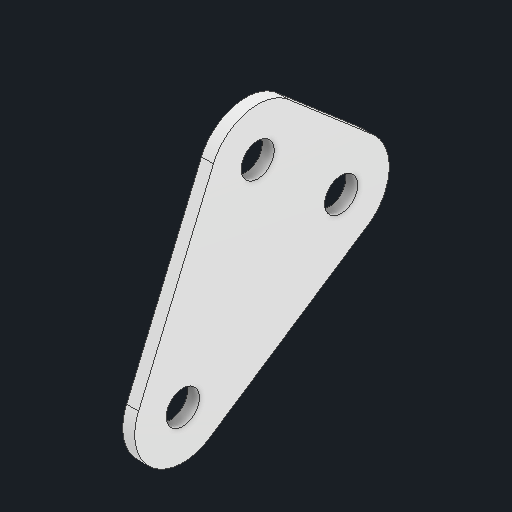
# Autodesk Inventor part: Conveyer Gusset
Saved by Autodesk Inventor 2025 (Build 290162000, 162)
## iProperties
Created: 2025-01-01
Part Number: Conveyer Gusset
Material: Acetal Resin, White
Document SubType Name: Modeling
Designer: Averey Ku
Density: 1.425 g/cm^3
Appearance: Smooth - White
Author: Averey Ku
Autodesk Inventor part; units mm, degrees
ref_plane "YZ Plane" through (0, 0, 0) normal (1, 0, 0) x (0, 1, 0)
ref_plane "XZ Plane" through (0, 0, 0) normal (0, 1, 0) x (-1, 0, 0)
ref_plane "XY Plane" through (0, 0, 0) normal (0, 0, 1) x (1, 0, 0)
sketch "Sketch1" plane through (0, 0, 0) normal (1, 0, 0) x (0, 1, 0)
  circle A0 centre (4.2685, -9.9057) radius 2.1844
  circle A1 centre (13.7537, 1.1357) radius 2.1844
  circle A2 centre (-9.6373, 11.0363) radius 2.1844
  arc A3 (18.5704, -3.0021) -> (16.2288, 6.9834) centre (13.7537, 1.1357) ccw
  arc A4 (-1.0214, -13.4183) -> (9.0853, -14.0435) centre (4.2685, -9.9057) ccw
  arc A5 (-7.1621, 16.884) -> (-14.9273, 7.5236) centre (-9.6373, 11.0363) ccw
  line L0 (-7.1621, 16.884) -> (16.2288, 6.9834)
  line L1 (-14.9273, 7.5236) -> (-1.0214, -13.4183)
  line L2 (18.5704, -3.0021) -> (9.0853, -14.0435)
  point P0 (0, 0)
  dimension "d0" = 12.7
  dimension "d1" = 12.7
  dimension "d2" = 12.7
  constraints: 6 centre point, 6 end point, 6 point on circle, 6 tangent, 3 coincident, 3 other
  measures "d0" diameter of A3
  measures "d1" diameter of A4
  measures "d2" diameter of A5
extrude "Extrusion1" add sketch "Sketch1" along normal blind 1.5875
body "Solid1"
